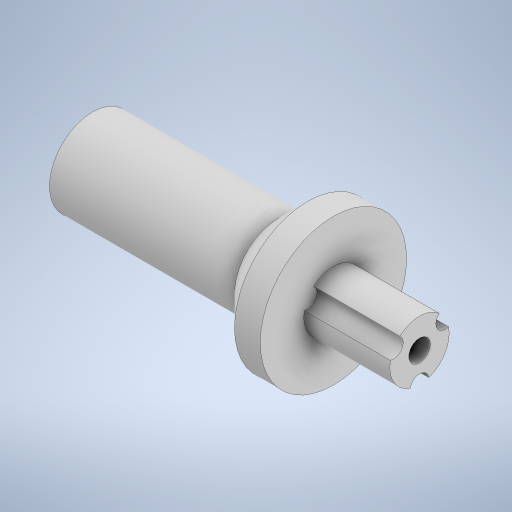
# Autodesk Inventor part: передача момента
Saved by Autodesk Inventor 2023 (Build 270158000, 158)
## iProperties
Created: 2023-04-09
Part Number: передача момента
Material: Типовые
Document SubType Name: Modeling
Designer: deryu
Density: 1 g/cm^3
Appearance: По умолчанию
Author: deryu
Autodesk Inventor part; units mm, degrees
ref_plane "YZ Plane" through (0, 0, 0) normal (1, 0, 0) x (0, 1, 0)
ref_plane "XZ Plane" through (0, 0, 0) normal (0, 1, 0) x (-1, 0, 0)
ref_plane "XY Plane" through (0, 0, 0) normal (0, 0, 1) x (1, 0, 0)
sketch "Эскиз1" plane through (0, 0, 0) normal (1, 0, 0) x (0, 1, 0)
  arc A0 (1.9, 1.7748) -> (1.9, -1.7748) centre (0, 0) ccw
  line L0 (0, 0) -> (1.9, 0)
  line L1 (1.9, 0) -> (1.9, -1.7748)
  line L2 (1.9, 0) -> (1.9, 1.7748)
  circle A1 centre (0, 0) radius 5
  dimension "d0" = 5.2
  dimension "d1" = 1.9
  dimension "d2" = 10
  constraints: 6 end point, 2 centre point, 2 coincident, 2 point on circle, 2 vertical, 1 horizontal
  measures "d0" diameter of A0
  measures "d1" distance of L0.start L0.end
  measures "d2" diameter of A1
extrude "Выдавливание1" add sketch "Эскиз1" along normal blind 25
sketch "Эскиз2" plane through (25, 0, 0) normal (1, 0, 0) x (0, 0, -1)
  circle A0 centre (0, 0) radius 3.45
  circle A1 centre (0, -3.45) radius 1.1
  circle A2 centre (2.9878, 1.725) radius 1.1
  circle A3 centre (-2.9878, 1.725) radius 1.1
  circle A4 centre (0, 0) radius 8.5
  point P0 (-2.293, 2.5778)
  point P1 (-3.3789, 0.6969)
  point P2 (-1.0859, -3.2746)
  point P3 (1.0859, -3.2746)
  point P4 (3.3789, 0.6969)
  point P5 (2.293, 2.5778)
  dimension "d5" = 6.9
  dimension "d6" = 2.2
  dimension "d9" = 360
  dimension "d13" = 17
  constraints: 4 centre point, 2 coincident, 10 other
  measures "d6" diameter of A1
  measures "d13" diameter of A4
extrude "Выдавливание2" add sketch "Эскиз2" along normal blind 13 contours A0 A1 A3 A2
sketch "Эскиз3" plane through (25, 0, 0) normal (1, 0, 0) x (0, 0, -1)
  circle A0 centre (0, 0) radius 8.5
  dimension "d14" = 17
  constraints: 1 centre point, 1 coincident
  measures "d14" diameter of A0
extrude "Выдавливание3" add sketch "Эскиз3" along normal blind 3
chamfer "Фаска1" distance 3.5 angle 45 1 edges at (25, -5, 0)
sketch "Эскиз4" plane through (38, 0, 0) normal (1, 0, 0) x (0, 0, -1)
  circle A0 centre (0, 0) radius 1.25
  dimension "d20" = 2.5
  constraints: 1 centre point, 1 coincident
  measures "d20" diameter of A0
extrude "Выдавливание4" cut sketch "Эскиз4" against normal through all
